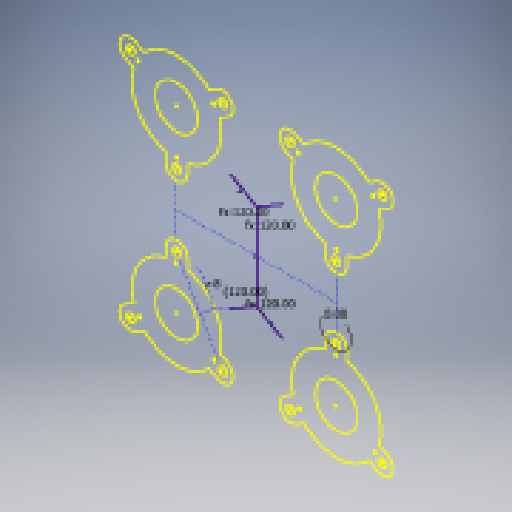
# Autodesk Inventor part: CE-7.1.1_RG
Saved by Autodesk Inventor 2024 (Build 280153000, 153)
## iProperties
Created: 2024-02-25
Part Number: CE-7.1.1_RG
Material: Generic
Document SubType Name: Modeling
Designer: Alex
Density: 1 g/cm^3
Appearance: Default
Author: Alex
Autodesk Inventor part; units mm, degrees
ref_plane "YZ Plane" through (0, 0, 0) normal (1, 0, 0) x (0, 1, 0)
ref_plane "XZ Plane" through (0, 0, 0) normal (0, 1, 0) x (-1, 0, 0)
ref_plane "Work Plane1" through (37.5, 37.5, -5.5) normal (0, 0, 1) x (0, 1, 0)
sketch "Sketch1" plane through (37.5, 37.5, -5.5) normal (0, 0, 1) x (0, 1, 0)
  circle A0 centre (14.4095, 57.5584) radius 0.75 projected
  circle A1 centre (14.4031, 93.082) radius 0.75 projected
  circle A2 centre (-15.9947, 74.8411) radius 0.75 projected
  circle A3 centre (16.9816, 96.6767) radius 2 projected
  circle A4 centre (16.9816, 53.3755) radius 2 projected
  circle A5 centre (-20.5184, 75.0261) radius 2 projected
  arc A6 (19.0756, 59.8532) -> (19.0367, 90.2363) centre (4.4816, 75.0261) ccw projected
  line L0 (10.3247, 54.8009) -> (12.6061, 50.8493) projected
  arc A7 (12.6061, 50.8493) -> (21.3571, 55.9016) centre (16.9816, 53.3755) ccw projected
  line L1 (21.3571, 55.9016) -> (19.0756, 59.8532) projected
  arc A8 (10.3765, 95.2363) -> (-15.9555, 80.0785) centre (4.4816, 75.0261) ccw projected
  line L2 (19.0367, 90.2363) -> (21.3117, 94.1767) projected
  arc A9 (21.3117, 94.1767) -> (12.6515, 99.1767) centre (16.9816, 96.6767) ccw projected
  line L3 (12.6515, 99.1767) -> (10.3765, 95.2363) projected
  arc A10 (-15.9555, 69.9737) -> (10.3247, 54.8009) centre (4.4816, 75.0261) ccw projected
  line L4 (-15.9555, 80.0785) -> (-20.5184, 80.0785) projected
  arc A11 (-20.5184, 80.0785) -> (-20.5184, 69.9737) centre (-20.5184, 75.0261) ccw projected
  line L5 (-20.5184, 69.9737) -> (-15.9555, 69.9737) projected
  circle A12 centre (4.4816, 75.0261) radius 10 projected
  circle A13 centre (14.4095, -17.4416) radius 0.75 projected
  circle A14 centre (14.4031, 18.082) radius 0.75 projected
  circle A15 centre (-15.9947, -0.1589) radius 0.75 projected
  circle A16 centre (16.9816, 21.6767) radius 2 projected
  circle A17 centre (16.9816, -21.6245) radius 2 projected
  circle A18 centre (-20.5184, 0.0261) radius 2 projected
  arc A19 (19.0756, -15.1468) -> (19.0367, 15.2363) centre (4.4816, 0.0261) ccw projected
  line L6 (10.3247, -20.1991) -> (12.6061, -24.1507) projected
  arc A20 (12.6061, -24.1507) -> (21.3571, -19.0984) centre (16.9816, -21.6245) ccw projected
  line L7 (21.3571, -19.0984) -> (19.0756, -15.1468) projected
  arc A21 (10.3765, 20.2363) -> (-15.9555, 5.0785) centre (4.4816, 0.0261) ccw projected
  line L8 (19.0367, 15.2363) -> (21.3117, 19.1767) projected
  arc A22 (21.3117, 19.1767) -> (12.6515, 24.1767) centre (16.9816, 21.6767) ccw projected
  line L9 (12.6515, 24.1767) -> (10.3765, 20.2363) projected
  arc A23 (-15.9555, -5.0263) -> (10.3247, -20.1991) centre (4.4816, 0.0261) ccw projected
  line L10 (-15.9555, 5.0785) -> (-20.5184, 5.0785) projected
  arc A24 (-20.5184, 5.0785) -> (-20.5184, -5.0263) centre (-20.5184, 0.0261) ccw projected
  line L11 (-20.5184, -5.0263) -> (-15.9555, -5.0263) projected
  circle A25 centre (4.4816, 0.0261) radius 10 projected
  circle A26 centre (-89.4095, 92.4416) radius 0.75 projected
  circle A27 centre (-89.4031, 56.918) radius 0.75 projected
  circle A28 centre (-59.0053, 75.1589) radius 0.75 projected
  circle A29 centre (-91.9816, 53.3233) radius 2 projected
  circle A30 centre (-91.9816, 96.6245) radius 2 projected
  circle A31 centre (-54.4816, 74.9739) radius 2 projected
  arc A32 (-94.0756, 90.1468) -> (-94.0367, 59.7637) centre (-79.4816, 74.9739) ccw projected
  line L12 (-85.3247, 95.1991) -> (-87.6061, 99.1507) projected
  arc A33 (-87.6061, 99.1507) -> (-96.3571, 94.0984) centre (-91.9816, 96.6245) ccw projected
  line L13 (-96.3571, 94.0984) -> (-94.0756, 90.1468) projected
  arc A34 (-85.3765, 54.7637) -> (-59.0445, 69.9215) centre (-79.4816, 74.9739) ccw projected
  line L14 (-94.0367, 59.7637) -> (-96.3117, 55.8233) projected
  arc A35 (-96.3117, 55.8233) -> (-87.6515, 50.8233) centre (-91.9816, 53.3233) ccw projected
  line L15 (-87.6515, 50.8233) -> (-85.3765, 54.7637) projected
  arc A36 (-59.0445, 80.0263) -> (-85.3247, 95.1991) centre (-79.4816, 74.9739) ccw projected
  line L16 (-59.0445, 69.9215) -> (-54.4816, 69.9215) projected
  arc A37 (-54.4816, 69.9215) -> (-54.4816, 80.0263) centre (-54.4816, 74.9739) ccw projected
  line L17 (-54.4816, 80.0263) -> (-59.0445, 80.0263) projected
  circle A38 centre (-79.4816, 74.9739) radius 10 projected
  circle A39 centre (-89.4095, 17.4416) radius 0.75 projected
  circle A40 centre (-89.4031, -18.082) radius 0.75 projected
  circle A41 centre (-59.0053, 0.1589) radius 0.75 projected
  circle A42 centre (-91.9816, -21.6767) radius 2 projected
  circle A43 centre (-91.9816, 21.6245) radius 2 projected
  circle A44 centre (-54.4816, -0.0261) radius 2 projected
  arc A45 (-94.0756, 15.1468) -> (-94.0367, -15.2363) centre (-79.4816, -0.0261) ccw projected
  line L18 (-85.3247, 20.1991) -> (-87.6061, 24.1507) projected
  arc A46 (-87.6061, 24.1507) -> (-96.3571, 19.0984) centre (-91.9816, 21.6245) ccw projected
  line L19 (-96.3571, 19.0984) -> (-94.0756, 15.1468) projected
  arc A47 (-85.3765, -20.2363) -> (-59.0445, -5.0785) centre (-79.4816, -0.0261) ccw projected
  line L20 (-94.0367, -15.2363) -> (-96.3117, -19.1767) projected
  arc A48 (-96.3117, -19.1767) -> (-87.6515, -24.1767) centre (-91.9816, -21.6767) ccw projected
  line L21 (-87.6515, -24.1767) -> (-85.3765, -20.2363) projected
  arc A49 (-59.0445, 5.0263) -> (-85.3247, 20.1991) centre (-79.4816, -0.0261) ccw projected
  line L22 (-59.0445, -5.0785) -> (-54.4816, -5.0785) projected
  arc A50 (-54.4816, -5.0785) -> (-54.4816, 5.0263) centre (-54.4816, -0.0261) ccw projected
  line L23 (-54.4816, 5.0263) -> (-59.0445, 5.0263) projected
  circle A51 centre (-79.4816, -0.0261) radius 10 projected
  line L24 (-49.4292, 74.9739) -> (-25.5705, 74.9739) construction
  line L25 (-49.4292, -0.0261) -> (-25.5705, -0.0261) construction
  line L26 (-49.4292, -0.0261) -> (-25.5705, -0.0261) construction
  line L27 (-91.9816, 53.3233) -> (-54.4816, 74.9739) construction
  line L28 (-73.2316, 64.1486) -> (-68.9554, 56.742) construction
  line L29 (-57.831, 37.4739) -> (-17.1688, 37.4739)
  line L30 (-68.9554, 56.742) -> (-55.4814, 64.5212) construction
  line L31 (-68.9554, 56.742) -> (-64.9554, 49.8138) construction
  line L32 (-64.9554, 49.8138) -> (-57.831, 37.4739)
  line L33 (-57.831, 37.4739) -> (-64.9554, 25.134)
  line L34 (-17.1688, 37.4739) -> (-10.0443, 25.134)
  line L35 (-17.1688, 37.4739) -> (-10.0443, 49.8138)
  line L36 (-37.4999, 74.9739) -> (-37.4999, -0.0261) construction
  point P0 (-37.4999, 37.4739)
  dimension "d1" = 0
  dimension "d2" = 8
  dimension "d3" = 120
  dimension "d4" = 120
  dimension "d5" = 120
  dimension "d6" = 120
  constraints: 26 end point, 5 midpoint, 4 equal length, 4 point on circle, 3 horizontal, 2 collinear, 2 perpendicular, 1 tangent
  measures "d1" distance between parallel lines of L25 L26
  measures "d2" distance from line of L31.end L30
  measures "d3" angle of L29 L32
  measures "d4" angle of L33 L29
  measures "d5" angle of L34 L29
  measures "d6" angle of L35 L29
sketch3d "3D Sketch1"
ref_plane "Work Plane2" through (-19.242, -31.4554, -5.5) normal (0.8660251, 0.5000006, 0) x (-0.5000006, 0.8660251, 0)
sketch3d "3D Sketch2"
ref_plane "Work Plane3" through (-19.0911, 31.8153, -5.5) normal (0.8410202, -0.5410036, 0) x (0.5410036, 0.8410202, 0)
sketch3d "3D Sketch3"
ref_plane "Work Plane4" through (19.242, 31.4554, -5.5) normal (-0.8643948, -0.5028137, 0) x (0.5028137, -0.8643948, 0)
sketch3d "3D Sketch4"
ref_plane "Work Plane5" through (19.0911, -31.8153, -5.5) normal (-0.8390936, 0.5439871, 0) x (-0.5439871, -0.8390936, 0)
sketch "Sketch2" plane through (0.0261, -20.331, -5.5) normal (0, 1, 0) x (-1, 0, 0)
  arc A0 (2, 0) -> (-2, 0) centre (0, 0) ccw
  line L0 (2, 0) -> (-2, 0)
  dimension "d7" = 2
  measures "d7" radius of A0
sweep "Sweep1" add profiles "Sketch2" path "Sketch1" path curves L29
sketch "Sketch3" plane through (0.0261, -24.331, -5.5) normal (0, 1, 0) x (-1, 0, 0)
  arc A0 (2, 0) -> (0, 2) centre (0, 0) ccw
  line L0 (0, 0) -> (0, 2)
  line L1 (0, 0) -> (2, 0)
  dimension "d11" = 2
  measures "d11" radius of A0
revolve "Revolution1" add sketch "Sketch3" angle 180 about axis through (0.0261, -24.331, -5.5) along (0, 0, 1)
sketch "Sketch4" plane through (0.0261, -20.331, -5.5) normal (0, 1, 0) x (-1, 0, 0)
  arc A0 (2, 0) -> (-2, 0) centre (0, 0) ccw
  line L0 (2, 0) -> (-2, 0)
  dimension "d13" = 2
  measures "d13" radius of A0
extrude "Extrusion1" add sketch "Sketch4" against normal blind 4
sketch "Sketch5" plane through (0.0261, 24.3312, -5.5) normal (0, 1, 0) x (-1, 0, 0)
  arc A0 (0, 2) -> (-2, 0) centre (0, 0) ccw
  line L0 (0, 0) -> (0, 2)
  line L1 (0, 0) -> (-2, 0)
  dimension "d17" = 2
  measures "d17" radius of A0
revolve "Revolution2" add sketch "Sketch5" angle 180 about axis through (0.0261, 24.3312, -5.5) along (0, 0, 1)
sketch "Sketch6" plane through (0.0261, 20.3312, -5.5) normal (0, 1, 0) x (-1, 0, 0)
  arc A0 (2, 0) -> (-2, 0) centre (0, 0) ccw
  line L0 (2, 0) -> (-2, 0)
  dimension "d19" = 2
  measures "d19" radius of A0
extrude "Extrusion2" add sketch "Sketch6" along normal blind 4
sketch "Sketch7" plane through (-12.3138, -27.4554, -5.5) normal (0.8660254, 0.5, 0) x (-0.5, 0.8660254, 0)
  arc A0 (2, 0) -> (-2, 0) centre (0, 0) ccw
  line L0 (2, 0) -> (-2, 0)
  dimension "d22" = 2
  measures "d22" radius of A0
sweep "Sweep2" add profiles "Sketch7" path "Sketch1" path curves L32
sketch "Sketch8" plane through (-14.0459, -28.4554, -5.5) normal (0.8660254, 0.5, 0) x (-0.5, 0.8660254, 0)
  arc A0 (2, 0) -> (0, 2) centre (0, 0) ccw
  line L0 (0, 0) -> (0, 2)
  line L1 (0, 0) -> (2, 0)
  dimension "d26" = 2
  measures "d26" radius of A0
revolve "Revolution3" add sketch "Sketch8" angle 180 about axis through (-14.0459, -28.4554, -5.5) along (0, 0, 1)
sketch "Sketch9" plane through (-12.3138, -27.4554, -5.5) normal (0.8660254, 0.5, 0) x (-0.5, 0.8660254, 0)
  arc A0 (2, 0) -> (-2, 0) centre (0, 0) ccw
  line L0 (2, 0) -> (-2, 0)
  dimension "d28" = 2
  measures "d28" radius of A0
extrude "Extrusion3" add sketch "Sketch9" against normal blind 2
sketch "Sketch10" plane through (0.0261, 20.3312, -5.5) normal (-0.8660254, 0.5, 0) x (-0.5, -0.8660254, 0)
  arc A0 (2, 0) -> (-2, 0) centre (0, 0) ccw
  line L0 (2, 0) -> (-2, 0)
  dimension "d31" = 2
  measures "d31" radius of A0
sweep "Sweep3" add profiles "Sketch10" path "Sketch1" path curves L35
sketch "Sketch11" plane through (-14.0459, 28.4557, -5.5) normal (-0.8660254, 0.5, 0) x (-0.5, -0.8660254, 0)
  arc A0 (0, 2) -> (-2, 0) centre (0, 0) ccw
  line L0 (0, 0) -> (0, 2)
  line L1 (0, 0) -> (-2, 0)
  dimension "d35" = 2
  measures "d35" radius of A0
revolve "Revolution4" add sketch "Sketch11" angle 180 about axis through (-14.0459, 28.4557, -5.5) along (0, 0, 1)
sketch "Sketch12" plane through (-12.3138, 27.4557, -5.5) normal (-0.8660254, 0.5, 0) x (-0.5, -0.8660254, 0)
  arc A0 (2, 0) -> (-2, 0) centre (0, 0) ccw
  line L0 (2, 0) -> (-2, 0)
  dimension "d37" = 2
  measures "d37" radius of A0
extrude "Extrusion4" add sketch "Sketch12" along normal blind 2
sketch "Sketch13" plane through (0.0261, 20.3312, -5.5) normal (0.8660254, 0.5, 0) x (-0.5, 0.8660254, 0)
  arc A0 (2, 0) -> (-2, 0) centre (0, 0) ccw
  line L0 (2, 0) -> (-2, 0)
  dimension "d40" = 2
  measures "d40" radius of A0
sweep "Sweep4" add profiles "Sketch13" path "Sketch1" path curves L34
sketch "Sketch14" plane through (14.0981, 28.4557, -5.5) normal (0.8660254, 0.5, 0) x (-0.5, 0.8660254, 0)
  arc A0 (0, 2) -> (-2, 0) centre (0, 0) ccw
  line L0 (0, 0) -> (0, 2)
  line L1 (0, 0) -> (-2, 0)
  dimension "d44" = 2
  measures "d44" radius of A0
revolve "Revolution5" add sketch "Sketch14" angle 180 about axis through (14.0981, 28.4557, -5.5) along (0, 0, 1)
sketch "Sketch15" plane through (12.366, 27.4557, -5.5) normal (0.8660254, 0.5, 0) x (-0.5, 0.8660254, 0)
  arc A0 (2, 0) -> (-2, 0) centre (0, 0) ccw
  line L0 (2, 0) -> (-2, 0)
  dimension "d46" = 2
  measures "d46" radius of A0
extrude "Extrusion5" add sketch "Sketch15" along normal blind 2
sketch "Sketch16" plane through (0.0261, -20.331, -5.5) normal (0.8660254, -0.5, 0) x (0.5, 0.8660254, 0)
  arc A0 (2, 0) -> (-2, 0) centre (0, 0) ccw
  line L0 (2, 0) -> (-2, 0)
  dimension "d49" = 2
  measures "d49" radius of A0
sweep "Sweep5" add profiles "Sketch16" path "Sketch1" path curves L33
sketch "Sketch17" plane through (14.0981, -28.4554, -5.5) normal (0.8660254, -0.5, 0) x (0.5, 0.8660254, 0)
  arc A0 (0, 2) -> (-2, 0) centre (0, 0) ccw
  line L0 (0, 0) -> (0, 2)
  line L1 (0, 0) -> (-2, 0)
  dimension "d1" = 0
  dimension "d2" = 8
  dimension "d3" = 120
  dimension "d4" = 120
  dimension "d5" = 120
  dimension "d6" = 120
  dimension "d53" = 2
  measures "d53" radius of A0
revolve "Revolution6" add sketch "Sketch17" angle 180 about axis through (14.0981, -28.4554, -5.5) along (0, 0, 1)
sketch "Sketch18" plane through (12.366, -27.4554, -5.5) normal (0.8660254, -0.5, 0) x (0.5, 0.8660254, 0)
  arc A0 (2, 0) -> (-2, 0) centre (0, 0) ccw
  line L0 (2, 0) -> (-2, 0)
  dimension "d55" = 2
  measures "d55" radius of A0
extrude "Extrusion6" add sketch "Sketch18" along normal blind 2
sketch "Sketch19" plane through (0.0261, -0.0926, -5.5) normal (0, 0, 1) x (1, 0, 0)
  circle A0 centre (0, 0) radius 5
  constraints: 1 centre point
extrude "Extrusion7" add sketch "Sketch19" against normal blind 8 draft 5
sketch "Sketch20" plane through (-18.376, -30.9554, -5.5) normal (0.8660251, 0.5000006, 0) x (-0.5000006, 0.8660251, 0)
  line L0 (-1, 0) -> (1, 0)
  line L1 (-0.9319, 1.3) -> (0.9319, 1.3)
  line L2 (-1, 0) -> (-0.9319, 1.3)
  line L3 (1, 0) -> (0.9319, 1.3)
  point P0 (0, 0)
  dimension "d61" = 2
  dimension "d62" = 1.3
  dimension "d63" = 87
  dimension "d64" = 87
  constraints: 8 end point, 1 horizontal, 1 midpoint
  measures "d61" distance of L0.start L0.end
  measures "d62" distance between parallel lines of L0 L1
  measures "d63" angle of L0 L2
  measures "d64" angle of L0 L3
sketch "Sketch21" plane through (-12.3138, -27.4554, -5.5) normal (0.8660251, 0.5000006, 0) x (-0.5000006, 0.8660251, 0)
  line L0 (-2, 0) -> (2, 0)
  line L1 (-1.8952, 2) -> (1.8952, 2)
  line L2 (-2, 0) -> (-1.8952, 2)
  line L3 (2, 0) -> (1.8952, 2)
  point P0 (0, 0)
  dimension "d65" = 4
  dimension "d66" = 2
  dimension "d67" = 87
  dimension "d68" = 87
  constraints: 8 end point, 1 horizontal, 1 midpoint
  measures "d65" distance of L0.start L0.end
  measures "d66" distance between parallel lines of L0 L1
  measures "d67" angle of L0 L2
  measures "d68" angle of L0 L3
loft "Loft1" add profiles "Sketch20", "Sketch21"
thicken "Thicken1" operation add thickness 1 both sides no extend neighbours no toward (-0.8660251, -0.5000006, 0) faces at (-18.2207, -31.2244, -5.0667)
sketch "Sketch22" plane through (-18.2501, 31.2743, -5.5) normal (0.8410202, -0.5410036, 0) x (0.5410036, 0.8410202, 0)
  line L0 (-1, 0) -> (1, 0)
  line L1 (-0.9319, 1.3) -> (0.9319, 1.3)
  line L2 (-1, 0) -> (-0.9319, 1.3)
  line L3 (1, 0) -> (0.9319, 1.3)
  point P0 (0, 0)
  dimension "d75" = 2
  dimension "d76" = 1.3
  dimension "d77" = 87
  dimension "d78" = 87
  constraints: 8 end point, 1 horizontal, 1 midpoint
  measures "d75" distance of L0.start L0.end
  measures "d76" distance between parallel lines of L0 L1
  measures "d77" angle of L0 L2
  measures "d78" angle of L0 L3
sketch "Sketch23" plane through (-12.3138, 27.4557, -5.5) normal (0.8410202, -0.5410036, 0) x (0.5410036, 0.8410202, 0)
  line L0 (-2, 0) -> (2, 0)
  line L1 (-1.8952, 2) -> (1.8952, 2)
  line L2 (-2, 0) -> (-1.8952, 2)
  line L3 (2, 0) -> (1.8952, 2)
  point P0 (0, 0)
  dimension "d79" = 4
  dimension "d80" = 2
  dimension "d81" = 87
  dimension "d82" = 87
  constraints: 8 end point, 1 horizontal, 1 midpoint
  measures "d79" distance of L0.start L0.end
  measures "d80" distance between parallel lines of L0 L1
  measures "d81" angle of L0 L2
  measures "d82" angle of L0 L3
loft "Loft2" add profiles "Sketch22", "Sketch23"
thicken "Thicken2" operation add thickness 1 both sides no extend neighbours no toward (-0.8410202, 0.5410036, 0) faces at (-18.4181, 31.0131, -5.0667)
sketch "Sketch24" plane through (18.3777, 30.9526, -5.5) normal (-0.8643948, -0.5028137, 0) x (0.5028137, -0.8643948, 0)
  line L0 (-1, 0) -> (1, 0)
  line L1 (-0.9319, 1.3) -> (0.9319, 1.3)
  line L2 (-1, 0) -> (-0.9319, 1.3)
  line L3 (1, 0) -> (0.9319, 1.3)
  point P0 (0, 0)
  dimension "d89" = 2
  dimension "d90" = 1.3
  dimension "d91" = 87
  dimension "d92" = 87
  constraints: 8 end point, 1 horizontal, 1 midpoint
  measures "d89" distance of L0.start L0.end
  measures "d90" distance between parallel lines of L0 L1
  measures "d91" angle of L0 L2
  measures "d92" angle of L0 L3
sketch "Sketch25" plane through (12.366, 27.4557, -5.5) normal (-0.8643948, -0.5028137, 0) x (0.5028137, -0.8643948, 0)
  line L0 (-2, 0) -> (2, 0)
  line L1 (-1.8952, 2) -> (1.8952, 2)
  line L2 (-2, 0) -> (-1.8952, 2)
  line L3 (2, 0) -> (1.8952, 2)
  point P0 (0, 0)
  dimension "d93" = 4
  dimension "d94" = 2
  dimension "d95" = 87
  dimension "d96" = 87
  constraints: 8 end point, 1 horizontal, 1 midpoint
  measures "d93" distance of L0.start L0.end
  measures "d94" distance between parallel lines of L0 L1
  measures "d95" angle of L0 L2
  measures "d96" angle of L0 L3
loft "Loft3" add profiles "Sketch24", "Sketch25"
thicken "Thicken3" operation add thickness 1 both sides no extend neighbours no toward (0.8643948, 0.5028137, 0) faces at (18.5338, 30.6841, -5.0667)
sketch "Sketch26" plane through (18.252, -31.2713, -5.5) normal (-0.8390936, 0.5439871, 0) x (-0.5439871, -0.8390936, 0)
  line L0 (-1, 0) -> (1, 0)
  line L1 (-0.9319, 1.3) -> (0.9319, 1.3)
  line L2 (-1, 0) -> (-0.9319, 1.3)
  line L3 (1, 0) -> (0.9319, 1.3)
  point P0 (0, 0)
  dimension "d103" = 2
  dimension "d104" = 1.3
  dimension "d105" = 87
  dimension "d106" = 87
  constraints: 8 end point, 1 horizontal, 1 midpoint
  measures "d103" distance of L0.start L0.end
  measures "d104" distance between parallel lines of L0 L1
  measures "d105" angle of L0 L2
  measures "d106" angle of L0 L3
sketch "Sketch27" plane through (12.366, -27.4554, -5.5) normal (-0.8390936, 0.5439871, 0) x (-0.5439871, -0.8390936, 0)
  line L0 (-2, 0) -> (2, 0)
  line L1 (-1.8952, 2) -> (1.8952, 2)
  line L2 (-2, 0) -> (-1.8952, 2)
  line L3 (2, 0) -> (1.8952, 2)
  point P0 (0, 0)
  dimension "d107" = 4
  dimension "d108" = 2
  dimension "d109" = 87
  dimension "d110" = 87
  constraints: 8 end point, 1 horizontal, 1 midpoint
  measures "d107" distance of L0.start L0.end
  measures "d108" distance between parallel lines of L0 L1
  measures "d109" angle of L0 L2
  measures "d110" angle of L0 L3
loft "Loft4" add profiles "Sketch26", "Sketch27"
thicken "Thicken4" operation add thickness 1 both sides no extend neighbours no toward (0.8390936, -0.5439871, 0) faces at (18.421, -31.0107, -5.0667)
equation "\"d4\" = d3"
equation "\"d5\" = d3"
equation "\"d6\" = d3"
equation "\"d64\" = d63"
equation "\"d68\" = d67"
equation "\"d78\" = d77"
equation "\"d82\" = d81"
equation "\"d92\" = d91"
equation "\"d96\" = d95"
equation "\"d106\" = d105"
equation "\"d110\" = d109"
body "Solid1"
